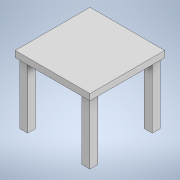
# Autodesk Inventor part: Tabl 12x12
Saved by Autodesk Inventor 2021 (Build 250183000, 183)
## iProperties
Created: 2021-02-17
Part Number: Tabl 12x12
Material: Generic
Document SubType Name: Modeling
Designer: david
Density: 1 g/cm^3
Appearance: Default
Author: david
Autodesk Inventor part; units mm, degrees
ref_plane "YZ Plane" through (0, 0, 0) normal (1, 0, 0) x (0, 1, 0)
ref_plane "XZ Plane" through (0, 0, 0) normal (0, 1, 0) x (-1, 0, 0)
ref_plane "XY Plane" through (0, 0, 0) normal (0, 0, 1) x (1, 0, 0)
sketch "Sketch1" plane through (0, 0, 0) normal (0, 1, 0) x (-1, 0, 0)
  line L0 (92.7652, 145.7739) -> (-212.0348, 145.7739)
  line L1 (-212.0348, 145.7739) -> (-212.0348, -159.0261)
  line L2 (-212.0348, -159.0261) -> (92.7652, -159.0261)
  line L3 (92.7652, -159.0261) -> (92.7652, 145.7739)
  point P0 (0, 0)
  dimension "d0" = 304.8
  dimension "d1" = 304.8
  constraints: 8 end point, 2 parallel, 1 horizontal, 1 perpendicular
  measures "d0" distance of L2.end L0.start
  measures "d1" distance of L1.end L2.end
extrude "Extrusion1" add sketch "Sketch1" along normal blind 25.4
sketch "Sketch2" plane through (0, 0, 0) normal (0, -1, 0) x (1, 0, 0)
  line L0 (199.3348, 133.0739) -> (166.6875, 133.0739)
  line L1 (166.6875, 133.0739) -> (166.6875, 101.6)
  line L2 (166.6875, 101.6) -> (199.3348, 101.6)
  line L3 (199.3348, 101.6) -> (199.3348, 133.0739)
  line L4 (212.0348, 145.7739) -> (212.0348, -159.0261) projected
  line L5 (-92.7652, 145.7739) -> (212.0348, 145.7739) projected
  line L6 (166.6875, -120.9261) -> (166.6875, -152.4)
  line L7 (199.3348, -120.9261) -> (166.6875, -120.9261)
  line L8 (199.3348, -152.4) -> (199.3348, -120.9261)
  line L9 (166.6875, -152.4) -> (199.3348, -152.4)
  line L10 (-87.3125, 133.0739) -> (-87.3125, 101.6)
  line L11 (-54.6652, 133.0739) -> (-87.3125, 133.0739)
  line L12 (-54.6652, 101.6) -> (-54.6652, 133.0739)
  line L13 (-87.3125, 101.6) -> (-54.6652, 101.6)
  line L14 (-87.3125, -120.9261) -> (-87.3125, -152.4)
  line L15 (-54.6652, -120.9261) -> (-87.3125, -120.9261)
  line L16 (-54.6652, -152.4) -> (-54.6652, -120.9261)
  line L17 (-87.3125, -152.4) -> (-54.6652, -152.4)
  point P0 (0, 0)
  dimension "d4" = 12.7
  dimension "d5" = 12.7
  dimension "d8" = 254
  dimension "d11" = 254
  constraints: 32 end point, 2 horizontal, 2 parallel, 1 perpendicular, 1 vertical, 24 other
  measures "d4" distance between parallel lines of L4 L3
  measures "d5" distance between parallel lines of L5 L0
  measures "d8" distance of L0.end L6.start
  measures "d11" distance of L0.end L10.start
extrude "Extrusion2" add sketch "Sketch2" along normal blind 254
body "Solid1"
